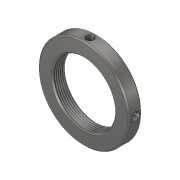
# Autodesk Inventor part: 05.01.002
Saved by Autodesk Inventor 2019.3 (Build 233278000, 278)
## iProperties
Created: 2018-07-09
Part Number: 05.01.002
Material: Сталь, углеродистая
Document SubType Name: Modeling
Designer: MSI-PC
Mass: 144.699 g
Surface Area: 74.4764 cm^2
Volume: 18.433 cm^3
Density: 7.85 g/cm^3
Appearance: С умеренной полировкой
Description: Гайка
Author: MSI-PC
Title: Гайка
Autodesk Inventor part; units mm, degrees
ref_plane "YZ Plane" through (0, 0, 0) normal (1, 0, 0) x (0, 1, 0)
ref_plane "XY Plane" through (0, 0, 0) normal (0, 0, 1) x (1, 0, 0)
sketch "Эскиз1" plane through (0, 0, 0) normal (0, 0, 1) x (1, 0, 0)
  circle A0 centre (0, 0) radius 34
  dimension "d0" = 68
  constraints: 1 centre point, 1 coincident
  measures "d0" diameter of A0
extrude "Выдавливание1" add sketch "Эскиз1" along normal mid plane 10
sketch "Эскиз2" plane through (0, 0, 5) normal (0, 0, 1) x (1, 0, 0)
  point P0 (0, 0)
  point P1 (0, 0)
  constraints: 1 coincident
hole "Отверстие1" at (0, 0, 5) direction (0, 0, -1) diameter 46.376 end through all thread size "M48x1.5" class "6H" standard "ISO Metric profile"
ref_plane "РабПлоскость1" through (0, 34, 0) normal (0, 1, 0) x (-1, 0, 0)
sketch "Эскиз3" plane through (0, 34, 0) normal (0, 1, 0) x (-1, 0, 0)
  point P0 (0, 0)
hole "Отверстие2" at (0, 34, 0) direction (0, -1, 0) diameter 6 depth 5 tip angle 118
pattern_circular "Круговой массив1" count 4 over 360 about axis through (0, 0, 0) along (0, 0, 1) of "Отверстие2"
chamfer "Фаска1" distance 1 angle 45 4 edges at (0, 23.188, 5) (0, 23.188, -5) (-34, 0, 5) (-34, 0, -5)
